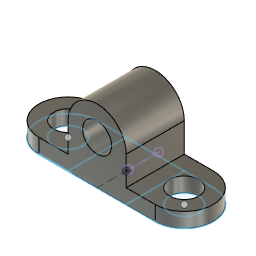
Piece-4 v3 (Autodesk Fusion 360 design; units mm, degrees)
Autodesk Fusion 360 part; units mm, degrees
sketch "Base" plane through (0, 0, 0) normal (0, 0, 1) x (1, 0, 0)
  line L0 (40, 20) -> (-40, 20)
  line L1 (-40, -20) -> (40, -20)
  line L2 (-20, 20) -> (-20, -20)
  line L3 (20, 20) -> (20, -20)
  circle A0 centre (-40, 0) radius 10
  circle A1 centre (40, 0) radius 10
  arc A2 (40, -20) -> (40, 20) centre (40, 0) ccw
  arc A3 (-40, 20) -> (-40, -20) centre (-40, 0) ccw
  line L4 (0, 20) -> (0, -20) construction
  line L5 (0, 1.75) -> (0, 22.5)
  dimension "d1" = 80
  dimension "d2" = 40
  dimension "d3" = 40
  dimension "d5" = 20
  dimension "d6" = 20
  dimension "d21" = 20
  constraint horizontal L0
  constraint parallel L0 L1
  constraint coincident L0 L2.start
  constraint coincident L1 L2.end
  constraint perpendicular L1 L2
  constraint coincident L0 L3.start
  constraint coincident L1 L3.end
  constraint perpendicular L1 L3
  constraint concentric A0 A3
  constraint concentric A1 A2
  constraint midpoint L0 L4.start
  constraint midpoint L1 L4.end
  constraint perpendicular L1 L4
  constraint collinear L4 L5
  measures "d1" distance of L1.start L1.end
  measures "d2" distance of L0.end L1.start
  measures "d3" distance of L2 L3
  measures "d5" diameter of A0
  measures "d6" diameter of A1
  measures "d21" radius of A3
extrude "Extrude1" add sketch "Base" along normal blind 10 contours L0 L1 L3 A2 | L0 L1 L2 A3 makes body 1 at (-23.3333, 0, 0) makes body 2 at (23.3333, 0, 0)
sketch "Round" plane through (0, 0, 0) normal (0, 1, 0) x (1, 0, 0)
  line L0 (-20, -30) -> (-20, 0)
  line L1 (-20, 0) -> (20, 0)
  line L2 (20, 0) -> (20, -30)
  line L3 (-40, 0) -> (40, 0)
  line L4 (0, -30) -> (0, 0) construction
  line L5 (0, -1.75) -> (0, -22.5) construction
  circle A0 centre (0, -30) radius 10
  arc A1 (-20, -30) -> (20, -30) centre (0, -30) ccw
  dimension "d11" = 30
  dimension "d12" = 40
  dimension "d13" = 20
  dimension "d14" = 40
  constraint vertical L0
  constraint horizontal L1
  constraint vertical L2
  constraint collinear L1 L3
  constraint midpoint L1 L4.end
  constraint collinear L4 L5
  constraint coincident L4.start A0.centre
  measures "d11" distance of L2.end L1.end
  measures "d12" distance of L2.end L0.start
  measures "d13" diameter of A0
  measures "d14" diameter of A1
extrude "Extrude3" add sketch "Round" along normal mid plane 40 bodies 1 2
named bodies: "Piece-4"
